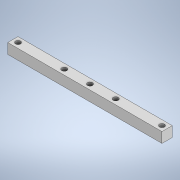
# Autodesk Inventor part: parallel_bar_long_v1
Saved by Autodesk Inventor 2022 (Build 260153000, 153)
## iProperties
Created: 2022-05-22
Part Number: parallel_bar_long_v1
Material: Generic
Document SubType Name: Modeling
Designer: kylem
Density: 1 g/cm^3
Appearance: Default
Author: kylem
Autodesk Inventor part; units mm, degrees
ref_plane "YZ Plane" through (0, 0, 0) normal (1, 0, 0) x (0, 1, 0)
ref_plane "XZ Plane" through (0, 0, 0) normal (0, 1, 0) x (-1, 0, 0)
ref_plane "XY Plane" through (0, 0, 0) normal (0, 0, 1) x (1, 0, 0)
sketch "Sketch1" plane through (0, 0, 0) normal (0, 1, 0) x (-1, 0, 0)
  line L0 (0, 0) -> (60, 0)
  line L1 (60, 0) -> (60, -4)
  line L2 (60, -4) -> (0, -4)
  line L3 (0, -4) -> (0, 0)
  dimension "d0" = 60
  dimension "d1" = 4
  constraints: 8 end point, 2 parallel, 1 horizontal, 1 perpendicular
  measures "d0" distance of L1.end L2.end
  measures "d1" distance of L0.end L1.end
extrude "Extrusion1" add sketch "Sketch1" along normal blind 4
sketch "Sketch2" plane through (0, 4, 0) normal (0, 1, 0) x (1, 0, 0)
  line L0 (0, 0) -> (0, 4) projected
  line L1 (0, 2) -> (-2, 2)
  circle A0 centre (-2, 2) radius 1
  line L2 (0, 4) -> (-60, 4) projected
  line L3 (-30, 4) -> (-30, 1.3223)
  circle A1 centre (-58, 2) radius 1
  dimension "d4" = 2
  dimension "d5" = 2
  constraints: 4 end point, 2 centre point, 2 midpoint, 1 coincident, 1 horizontal, 1 symmetric about line, 1 vertical, 1 other
  measures "d4" distance of L1.start L1.end
  measures "d5" diameter of A0
extrude "Extrusion2" cut sketch "Sketch2" against normal blind 4
sketch "Sketch3" plane through (0, 4, 0) normal (0, 1, 0) x (1, 0, 0)
  line L0 (0, 0) -> (0, 4) projected
  line L1 (0, 2) -> (-60, 2)
  line L2 (-60, 4) -> (-60, 0) projected
  circle A0 centre (-30, 2) radius 1
  circle A1 centre (-20, 2) radius 1
  circle A2 centre (-40, 2) radius 1
  circle A3 centre (-30, 2) radius 1
  dimension "d8" = 2
  dimension "d13" = 10
  dimension "d16" = 10
  constraints: 4 centre point, 3 midpoint, 2 end point, 2 horizontal, 6 other
  measures "d8" diameter of A0
  measures "d13" distance of A0.centre A1.centre
  measures "d16" distance of A0.centre A2.centre
extrude "Extrusion3" cut sketch "Sketch3" against normal blind 10 contours A0 L1 | L1 A0
extrude "Extrusion4" cut sketch "Sketch3" against normal blind 10 contours A1 L1 | L1 A1 | A2 L1 | L1 A2
body "Solid1"
